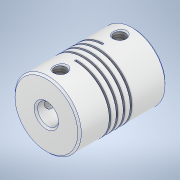
# Autodesk Inventor part: Wellenkupplung
Saved by Autodesk Inventor 2020 (Build 240168000, 168)
## iProperties
Created: 2021-10-17
Part Number: Wellenkupplung
Material: Aluminium 6061
Document SubType Name: Modeling
Designer: N. Vielberth
Density: 2.7 g/cm^3
Appearance: Aluminium - flach
Author: N. Vielberth
Autodesk Inventor part; units mm, degrees
ref_plane "YZ Plane" through (0, 0, 0) normal (1, 0, 0) x (0, 1, 0)
ref_plane "XY Plane" through (0, 0, 0) normal (0, 0, 1) x (1, 0, 0)
sketch "Skizze1" plane through (0, 0, 0) normal (0, 0, 1) x (1, 0, 0)
  circle A0 centre (0, 0) radius 9.5
  circle A1 centre (0, 0) radius 4
  dimension "d0" = 19
  dimension "d1" = 8
  constraints: 2 centre point, 2 coincident
  measures "d0" diameter of A0
  measures "d1" diameter of A1
extrude "Extrusion1" add sketch "Skizze1" along normal blind 25
sketch "Skizze2" plane through (0, 0, 25) normal (0, 0, 1) x (1, 0, 0)
  circle A0 centre (0, 0) radius 3
  circle A1 centre (0, 0) radius 4 projected
  dimension "d4" = 6
  constraints: 1 centre point, 1 coincident
  measures "d4" diameter of A0
extrude "Extrusion2" add sketch "Skizze2" against normal blind 10
sketch "Skizze3" plane through (0, 0, 0) normal (1, 0, 0) x (0, 1, 0)
  line L0 (10.275, 17) -> (1.3311, 17)
  line L1 (1.3311, 17) -> (1.3311, 16.5)
  line L2 (1.3311, 16.5) -> (10.275, 16.5)
  line L3 (10.275, 16.5) -> (10.275, 17)
  line L4 (9.5, 25) -> (-9.5, 25) projected
  point P0 (0, 0)
  dimension "d7" = 0.5
  dimension "d8" = 8
  constraints: 8 end point, 2 parallel, 1 horizontal, 1 perpendicular
  measures "d7" distance of L2.end L0.start
  measures "d8" distance between parallel lines of L0 L4
coil "Spirale1" sketch "Skizze3" operation cut axis through (0, 0, -10) along (0, 0, -1) pitch 2 turns 4 hand right
ref_plane "Arbeitsebene1" through (0, 9.5, 0) normal (0, 1, 0) x (-1, 0, 0)
sketch "Skizze4" plane through (0, 9.5, 0) normal (0, 1, 0) x (-1, 0, 0)
  line L0 (9.5, 25) -> (-9.5, 25) projected
  line L1 (9.5, 0) -> (-9.5, 0) projected
  line L2 (0, 0) -> (0, 29.039)
  point P0 (0, 21)
  point P1 (0, 4)
  dimension "d17" = 4
  dimension "d18" = 4
  constraints: 2 end point, 2 point on line, 1 vertical
  measures "d17" distance from line of L0 point (0, 21)
  measures "d18" distance from line of L1 point (0, 4)
hole "Bohrung1" at (0, 9.5, 21) at (0, 9.5, 4) direction (0, -1, 0) diameter 3.242 depth 11.8 tip angle 140 countersink diameter 4 countersink angle 90 thread size "M4x0.7" class "6H" standard "ISO Metric profile"
pattern_circular "Runde Anordnung1" count 2 over 90 about axis through (0, 0, 0) along (0, 0, 1) of "Bohrung1"
chamfer "Fase1" distance 0.5 angle 45 4 edges at (-9.5, 0, 25) (-9.5, 0, 0) (-3, 0, 25) (-4, 0, 0)
